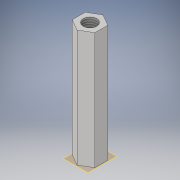
# Autodesk Inventor part: abstandshalter_26mm
Saved by Autodesk Inventor 2019 (Build 230136000, 136)
## iProperties
Created: 2021-05-27
Part Number: abstandshalter_26mm
Material: Generisch
Document SubType Name: Modeling
Designer: Lukas
Density: 1 g/cm^3
Appearance: Vorgabe
Author: Lukas
Autodesk Inventor part; units mm, degrees
ref_plane "YZ Plane" through (0, 0, 0) normal (1, 0, 0) x (0, 1, 0)
ref_plane "XY Plane" through (0, 0, 0) normal (0, 0, 1) x (1, 0, 0)
sketch "Skizze1" plane through (0, 0, 0) normal (0, 1, 0) x (-1, 0, 0)
  line L0 (0, 0) -> (0, -2.8868)
  line L1 (0, -2.8868) -> (-2.5, -4.3301)
  line L2 (-2.5, -4.3301) -> (-5, -2.8868)
  line L3 (-5, -2.8868) -> (-5, 0)
  line L4 (-5, 0) -> (-2.5, 1.4434)
  line L5 (-2.5, 1.4434) -> (0, 0)
  dimension "d2" = 120
  dimension "d4" = 120
  dimension "d6" = 120
  dimension "d8" = 120
  dimension "d11" = 5
  dimension "d12" = 5
  dimension "d13" = 5
  constraints: 12 end point, 2 parallel, 1 coincident, 1 equal length, 1 vertical
  measures "d2" angle of L0 L1
  measures "d4" angle of L1 L2
  measures "d6" angle of L2 L3
  measures "d8" angle of L3 L4
  measures "d11" distance between parallel lines of L3 L0
  measures "d12" distance between parallel lines of L5 L2
  measures "d13" distance between parallel lines of L1 L4
extrude "Extrusion1" add sketch "Skizze1" along normal blind 26
sketch "Skizze2" plane through (0, 26, 0) normal (0, 1, 0) x (1, 0, 0)
  line L0 (0, 2.8868) -> (0, 0) projected
  line L1 (5, 0) -> (5, 2.8868) projected
  line L2 (0, 0) -> (5, 2.8868) construction
  line L3 (0, 2.8868) -> (5, 0) construction
  point P0 (2.5, 1.4434)
  constraints: 4 end point, 1 midpoint
hole "Bohrung1" at (2.5, 26, -1.4434) direction (0, -1, 0) diameter 3 end through all
thread "Gewinde1" size "M3x0.5" class "6H" standard "ANSI Metric M Profile" full length
